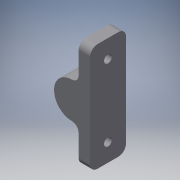
# Autodesk Inventor part: NASA-20-ARM-BR-01
Saved by Autodesk Inventor 2019 (Build 230136000, 136)
## iProperties
Created: 2019-09-08
Part Number: NASA-20-ARM-BR-01
Material: Generic
Document SubType Name: Modeling
Designer: Rick Szalay
Density: 1 g/cm^3
Appearance: Default
Author: Rick Szalay
Autodesk Inventor part; units mm, degrees
ref_plane "YZ Plane" through (0, 0, 0) normal (1, 0, 0) x (0, 1, 0)
ref_plane "XZ Plane" through (0, 0, 0) normal (0, 1, 0) x (-1, 0, 0)
ref_plane "XY Plane" through (0, 0, 0) normal (0, 0, 1) x (1, 0, 0)
sketch "Sketch1" plane through (0, 0, 0) normal (0, 0, 1) x (1, 0, 0)
  line L0 (5.475, -45) -> (15, -45)
  line L1 (15, -45) -> (15, 45)
  line L2 (15, 45) -> (5.475, 45)
  line L3 (5.475, -45) -> (15, 45) construction
  line L4 (15, -45) -> (5.475, 45) construction
  arc A0 (0, 15) -> (5.475, 20.475) centre (0, 20.475) ccw
  line L5 (5.475, 0) -> (15, 0) construction
  arc A1 (5.475, -20.475) -> (0, -15) centre (0, -20.475) ccw
  line L6 (5.475, 45) -> (5.475, 20.475)
  line L7 (5.475, -20.475) -> (5.475, -45)
  arc A2 (0, 15) -> (0, -15) centre (0, 0) ccw
  point P0 (10.2375, 0)
  point P1 (10.2375, 0)
  dimension "d1" = 90
  dimension "d2" = 9.525
  dimension "d3" = 15
  constraints: 16 end point, 6 point on circle, 4 midpoint, 4 tangent, 3 centre point, 3 parallel, 3 symmetric about line, 1 coincident, 1 horizontal, 1 horizontal alignment, 1 perpendicular, 1 vertical alignment, 1 other
  measures "d1" distance of L0.end L1.end
  measures "d2" distance of L1.end L2.end
  measures "d3" radius of A2
extrude "Extrusion1" add sketch "Sketch1" along normal blind 30
sketch "Sketch2" plane through (5.475, 20.475, 0) normal (-1, 0, 0) x (0, 0, 1)
  line L0 (0, -65.475) -> (30, -65.475) projected
  line L1 (0, 24.525) -> (30, 24.525) projected
  point P0 (0, -20.475)
  point P1 (15, 9.525)
  point P2 (15, -50.475)
  point P3 (15, -65.475)
  dimension "d6" = 15
  dimension "d7" = 15
  constraints: 2 vertical alignment, 1 midpoint
  measures "d6" distance from line of L1 point (15, 9.525)
  measures "d7" distance from line of L0 point (15, -50.475)
hole "Hole1" at (5.475, 30, 15) at (5.475, -30, 15) direction (1, 0, 0) diameter 6.604 end through all counterbore diameter 18.0086 counterbore depth 4.8006 clearance for "Hex Head Cap Screw DIN EN 24017" size "M6" standard "DIN"
fillet "Fillet1" radius 6.35 4 edges at (10.2375, -45, 30) (10.2375, 45, 30) (10.2375, 45, 0) (10.2375, -45, 0)
body "Solid1"
